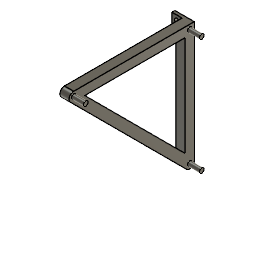
Pulley Assembly (Autodesk Fusion 360 archive; units mm, degrees)
design "Left support for pulley"
part number: 2026-04-03-14-57-29-841
Autodesk Fusion 360 part; units mm, degrees
sketch "Sketch1" plane through (0, 0, 0) normal (1, 0, 0) x (0, 1, 0)
  line L0 (171.704, 12.7) -> (-171.704, 12.7)
  line L1 (-171.704, 12.7) -> (-171.704, -12.7)
  line L2 (-171.704, -12.7) -> (171.704, -12.7)
  line L3 (171.704, -12.7) -> (171.704, 12.7)
  line L4 (171.704, 12.7) -> (-171.704, -12.7) construction
  line L5 (-171.704, 12.7) -> (171.704, -12.7) construction
  circle A0 centre (-159.004, 0) radius 12.7
  line L6 (171.704, -12.7) -> (146.304, -12.7)
  line L7 (146.304, -12.7) -> (146.304, -330.708)
  line L8 (146.304, -330.708) -> (171.704, -330.708)
  line L9 (171.704, -330.708) -> (171.704, -12.7)
  circle A1 centre (159.004, -318.008) radius 12.7
  line L10 (150.0237, -326.9883) -> (-167.9843, -8.9803)
  line L11 (150.0237, -326.9883) -> (167.9843, -309.0277)
  line L12 (150.0237, -326.9883) -> (175.4237, -326.9883) construction
  line L13 (167.9843, -309.0277) -> (-150.0237, 8.9803)
  dimension "d1" = 343.408
  dimension "d2" = 25.4
  dimension "d3" = 25.4
  dimension "d4" = 25.4
  dimension "d5" = 318.008
  dimension "d6" = 25.4
  dimension "d7" = 25.4
  dimension "d8" = 45
  constraint horizontal L0
  constraint perpendicular L0 L1
  constraint parallel L0 L2
  constraint parallel L1 L3
  constraint coincident L4 origin
  constraint coincident L5 origin
  constraint tangent L1 A0
  constraint tangent L0 A0
  constraint horizontal L6
  constraint vertical L7
  constraint horizontal L8
  constraint vertical L9
  constraint tangent L8 A1
  constraint tangent L9 A1
  constraint coincident A1 L10.start
  constraint coincident A0 L10.end
  constraint tangent A0 L10
  constraint tangent A1 L10
  constraint horizontal L12
  constraint coincident A0 L13.end
  constraint tangent A0 L13
  measures "d1" distance of L1.end L2.end
  measures "d2" distance of L0.end L1.end
  measures "d3" diameter of A0
  measures "d4" distance of L2.end L6.end
  measures "d5" distance of L2.end L8.end
  measures "d6" diameter of A1
  measures "d7" distance of L10.start L11.end
  measures "d8" angle of L11 L12
extrude "Extrude1" add sketch "Sketch1" along normal blind 25.4 contours L0 L2 L3 A0 L6 L13 | A0 | L2 L6 L7 L9 A1 L13 | L2 A0 L13 | A1 L11 | L2 L7 L10 L13 | L2 A0 L10 | L7 A1 L13 | A1 L11 | L7 A1 L10
sketch "Sketch2" plane through (0, 0, 0) normal (-1, 0, 0) x (0, -1, 0)
  line L0 (-146.304, -12.7) -> (128.3435, -12.7)
  line L1 (128.3435, -12.7) -> (-146.304, -287.3475)
  line L2 (-146.304, -287.3475) -> (-146.304, -12.7)
  line L3 (-171.704, 12.7) -> (-171.704, -318.008)
  arc A0 (-171.704, -318.008) -> (-150.0237, -326.9883) centre (-159.004, -318.008) ccw
  line L4 (-150.0237, -326.9883) -> (167.9843, -8.9803)
  arc A1 (167.9843, -8.9803) -> (159.004, 12.7) centre (159.004, 0) ccw
  line L5 (159.004, 12.7) -> (-171.704, 12.7)
  line L6 (-171.704, 12.7) -> (-163.322, 12.7)
  line L7 (-163.322, 12.7) -> (-163.322, -15.24)
  line L8 (-163.322, -15.24) -> (-171.704, -15.24)
  line L9 (-171.704, -15.24) -> (-171.704, 12.7)
  dimension "d11" = 8.382
  dimension "d12" = 27.94
  constraint horizontal L6
  constraint vertical L7
  constraint horizontal L8
  constraint vertical L9
  constraint coincident L3.start L5.end
  measures "d11" distance of L3.start L6.end
  measures "d12" distance of L3.start L8.end
extrude "Extrude2" add sketch "Sketch2" along normal blind 27.94 contours L3 L5 L6 L7 L8 L9
sketch "Sketch3" plane through (0, 163.322, 0) normal (0, -1, 0) x (1, 0, 0)
  line L0 (0, -15.24) -> (0, 12.7)
  line L1 (0, 12.7) -> (-27.94, 12.7)
  line L2 (-27.94, 12.7) -> (-27.94, -15.24)
  line L3 (-27.94, -15.24) -> (0, -15.24)
  circle A0 centre (-13.97, -1.27) radius 6.35
  dimension "d15" = 12.7
  measures "d15" diameter of A0
extrude "Extrude3" cut sketch "Sketch3" against normal blind 8.382 contours A0
sketch "Sketch4" plane through (25.4, 0, 0) normal (1, 0, 0) x (0, 1, 0)
  line L0 (-128.3435, -12.7) -> (146.304, -12.7)
  line L1 (146.304, -12.7) -> (146.304, -287.3475)
  line L2 (146.304, -287.3475) -> (-128.3435, -12.7)
  line L3 (171.704, -318.008) -> (171.704, 12.7)
  line L4 (171.704, 12.7) -> (-159.004, 12.7)
  arc A0 (-159.004, 12.7) -> (-167.9843, -8.9803) centre (-159.004, 0) ccw
  line L5 (-167.9843, -8.9803) -> (150.0237, -326.9883)
  arc A1 (150.0237, -326.9883) -> (171.704, -318.008) centre (159.004, -318.008) ccw
  circle A2 centre (-159.004, 0) radius 6.2865
  dimension "d18" = 12.573
  constraint concentric A0 A2
  measures "d18" diameter of A2
extrude "Extrude4" add sketch "Sketch4" along normal blind 33.02 contours A2
sketch "Sketch5" plane through (25.4, 0, 0) normal (1, 0, 0) x (0, 1, 0)
  circle A0 centre (-159.004, 0) radius 6.2865
  line L0 (-128.3435, -12.7) -> (146.304, -12.7)
  line L1 (146.304, -287.3475) -> (-128.3435, -12.7)
  line L2 (171.704, -318.008) -> (171.704, 12.7)
  line L3 (171.704, 12.7) -> (-159.004, 12.7)
  arc A1 (-159.004, 12.7) -> (-167.9843, -8.9803) centre (-159.004, 0) ccw
  line L4 (-167.9843, -8.9803) -> (150.0237, -326.9883)
  arc A2 (150.0237, -326.9883) -> (171.704, -318.008) centre (159.004, -318.008) ccw
  circle A3 centre (159.004, -318.008) radius 6.35
  dimension "d21" = 12.7
  constraint concentric A2 A3
  measures "d21" diameter of A3
extrude "Extrude5" add sketch "Sketch5" along normal blind 33.02 contours A3
sketch "Sketch6" plane through (25.4, 0, 0) normal (1, 0, 0) x (0, 1, 0)
  circle A0 centre (159.004, -318.008) radius 6.35
  circle A1 centre (-159.004, 0) radius 6.2865
  line L0 (-128.3435, -12.7) -> (146.304, -12.7)
  line L1 (146.304, -12.7) -> (146.304, -287.3475)
  line L2 (146.304, -287.3475) -> (-128.3435, -12.7)
  line L3 (171.704, -318.008) -> (171.704, 12.7)
  line L4 (171.704, 12.7) -> (-159.004, 12.7)
  arc A2 (-159.004, 12.7) -> (-167.9843, -8.9803) centre (-159.004, 0) ccw
  line L5 (-167.9843, -8.9803) -> (150.0237, -326.9883)
  arc A3 (150.0237, -326.9883) -> (171.704, -318.008) centre (159.004, -318.008) ccw
  line L6 (146.304, -12.7) -> (171.704, -12.7)
  line L7 (171.704, -12.7) -> (171.704, 12.7)
  line L8 (171.704, 12.7) -> (146.304, 12.7)
  line L9 (146.304, 12.7) -> (146.304, -12.7)
  circle A4 centre (159.004, 0) radius 6.35
  dimension "d24" = 12.7
  constraint horizontal L6
  constraint vertical L7
  constraint horizontal L8
  constraint vertical L9
  constraint coincident L3.end L4.start
  constraint coincident L0.end L1.start
  measures "d24" diameter of A4
extrude "Extrude6" add sketch "Sketch6" along normal blind 33.02 contours A4

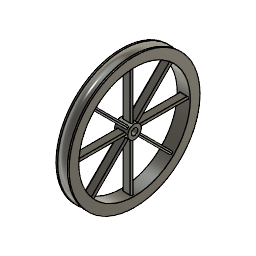
design "Pulley for the handle"
part number: 2026-04-03-13-48-15-446
Autodesk Fusion 360 part; units mm, degrees
sketch "Sketch1" plane through (0, 0, 0) normal (1, 0, 0) x (0, 1, 0)
  circle A0 centre (0, 0) radius 127
  circle A1 centre (0, 0) radius 107.95
  circle A2 centre (0, 0) radius 13.1264
  line L0 (2.8393, 12.8157) -> (2.8393, 107.9127)
  line L1 (-2.7344, 107.9154) -> (-2.7344, 12.8385)
  dimension "d1" = 254
  dimension "d2" = 215.9
  constraint coincident A0.centre A1.centre
  constraint coincident A2 L0.start
  constraint coincident A1 L0.end
  constraint vertical L0
  constraint coincident A1 L1.start
  constraint coincident A2 L1.end
  constraint parallel L0 L1
  measures "d1" diameter of A0
  measures "d2" diameter of A1
extrude "Extrude1" add sketch "Sketch1" along normal blind 19.05 contours A1 A2 L0 L1 picked at (0.3629, 44.7105) makes body 1
pattern_circular "C-Pattern1" count 8 over 360 about axis through (1.75, 0, 0) along (1, 0, 0) of bodies 1 makes body 2 at (6.35, -29.4689, 33.4843) makes body 3 at (12.7, -44.5147, 2.8393) makes body 4 at (6.35, -33.4843, -29.4689) makes body 5 at (12.7, -2.8393, -44.5147) makes body 6 at (6.35, 29.4689, -33.4843) makes body 7 at (12.7, 44.5147, -2.8393) makes body 8 at (6.35, 33.4843, 29.4689)
move_body "Move1" bodies 3 2 4 1 8 5 6 7 to x (1, 0, 0) y (0, 1, 0) z (0, 0, 1) at (3.175, 0, 0)
sketch "Sketch2" plane through (0, 0, 0) normal (1, 0, 0) x (0, 1, 0)
  circle A0 centre (0, 0) radius 13.2274
  circle A1 centre (0, 0) radius 107.95
  circle A2 centre (0, 0) radius 127
  constraint coincident A0.centre A1.centre
  constraint concentric A0 A1
  constraint concentric A1 A2
extrude "Extrude2" add sketch "Sketch2" along normal blind 25.4 bodies 1 2 3 4 5 6 7 8
sketch "Sketch3" plane through (0, 0, 0) normal (-1, 0, 0) x (0, -1, 0)
  circle A0 centre (0, 0) radius 13.2274
  circle A1 centre (0, 0) radius 6.35
  constraint concentric A0 A1
extrude "Extrude3" cut sketch "Sketch3" against normal blind 25.4 contours A1 bodies 1
sketch "Sketch4" plane through (0, 0, 0) normal (0, 1, 0) x (1, 0, 0)
  circle A0 centre (12.7, -127) radius 9.525
  dimension "d11" = 19.05
  measures "d11" diameter of A0
sketch "Sketch5" plane through (0, 0, 0) normal (1, 0, 0) x (0, 1, 0)
  circle A0 centre (0, 0) radius 127
  constraint coincident A0.centre origin
sweep "Sweep1" cut profiles "Sketch4" path "Sketch5" along A0 section 1 bodies 1
fillet "Fillet1" radius 2.7864 4 edges at (22.225, 2.8393, 60.4159) (22.225, -2.7344, 60.4285) (3.175, -2.7344, 60.4285) (3.175, 2.8393, 60.4159) on bodies 1
fillet "Fillet2" radius 2.7864 28 edges at (3.175, -44.6629, 40.7959) (3.175, -40.7127, 44.7282) (22.225, -40.7127, 44.7282) (22.225, -44.6629, 40.7959) (3.175, -60.4285, -2.7344) (22.225, -60.4159, 2.8393) (3.175, -60.4159, 2.8393) (22.225, -60.4285, -2.7344) (22.225, -44.7282, -40.7127) (3.175, -44.7282, -40.7127) (22.225, -40.7959, -44.6629) (3.175, -40.7959, -44.6629) (22.225, -2.8393, -60.4159) (22.225, 2.7344, -60.4285) (3.175, -2.8393, -60.4159) (3.175, 2.7344, -60.4285) (22.225, 40.7127, -44.7282) (22.225, 44.6629, -40.7959) (3.175, 40.7127, -44.7282) (3.175, 44.6629, -40.7959) (22.225, 60.4159, -2.8393) (22.225, 60.4285, 2.7344) (3.175, 60.4159, -2.8393) (3.175, 60.4285, 2.7344) (22.225, 40.7959, 44.6629) (22.225, 44.7282, 40.7127) (3.175, 40.7959, 44.6629) (3.175, 44.7282, 40.7127) on bodies 1

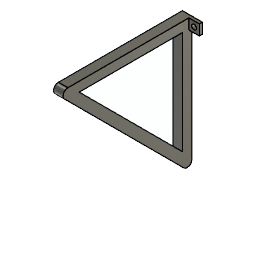
design "Right Support for Pulley"
part number: 2026-04-03-13-47-48-365
Autodesk Fusion 360 part; units mm, degrees
sketch "Sketch1" plane through (0, 0, 0) normal (1, 0, 0) x (0, 1, 0)
  line L0 (171.704, 12.7) -> (-171.704, 12.7)
  line L1 (-171.704, 12.7) -> (-171.704, -12.7)
  line L2 (-171.704, -12.7) -> (171.704, -12.7)
  line L3 (171.704, -12.7) -> (171.704, 12.7)
  line L4 (171.704, 12.7) -> (-171.704, -12.7) construction
  line L5 (-171.704, 12.7) -> (171.704, -12.7) construction
  circle A0 centre (-159.004, 0) radius 12.7
  line L6 (171.704, -12.7) -> (146.304, -12.7)
  line L7 (146.304, -12.7) -> (146.304, -330.708)
  line L8 (146.304, -330.708) -> (171.704, -330.708)
  line L9 (171.704, -330.708) -> (171.704, -12.7)
  circle A1 centre (159.004, -318.008) radius 12.7
  line L10 (-171.704, -5.2605) -> (150.0237, -326.9883)
  line L11 (-171.704, -5.2605) -> (-153.7435, 12.7)
  line L12 (-171.704, -5.2605) -> (-146.304, -5.2605) construction
  line L13 (-153.7435, 12.7) -> (170.7899, -311.8334)
  dimension "d1" = 343.408
  dimension "d2" = 25.4
  dimension "d3" = 25.4
  dimension "d4" = 318.008
  dimension "d5" = 25.4
  dimension "d6" = 45
  dimension "d7" = 25.4
  constraint horizontal L0
  constraint perpendicular L0 L1
  constraint parallel L0 L2
  constraint parallel L1 L3
  constraint coincident L4 origin
  constraint coincident L5 origin
  constraint tangent L1 A0
  constraint tangent L0 A0
  constraint horizontal L6
  constraint vertical L7
  constraint horizontal L8
  constraint vertical L9
  constraint tangent L8 A1
  constraint tangent L9 A1
  constraint coincident L1 L10.start
  constraint coincident A1 L10.end
  constraint tangent A1 L10
  constraint horizontal L12
  constraint perpendicular L10 L11
  constraint tangent A1 L13
  measures "d1" distance of L1.end L2.end
  measures "d2" distance of L0.end L1.end
  measures "d3" distance of L2.end L6.end
  measures "d4" distance of L2.end L8.end
  measures "d5" diameter of A1
  measures "d6" angle of L11 L12
  measures "d7" distance of L10.start L11.end
extrude "Extrude1" add sketch "Sketch1" along normal blind 25.4 contours L0 L2 L3 L6 L13 | L0 A0 L11 | A0 L11 L13 | L2 L6 L7 L9 A1 L13 | A0 L11 | A0 L11 | L2 A0 L13 | A1 | L2 L7 L10 L13 | L7 A1 L13 | L2 A0 L10 | L7 A1 L10
sketch "Sketch2" plane through (25.4, 0, 0) normal (1, 0, 0) x (0, 1, 0)
  line L0 (146.304, -287.3475) -> (-128.3435, -12.7)
  line L1 (-128.3435, -12.7) -> (146.304, -12.7)
  line L2 (146.304, -12.7) -> (146.304, -287.3475)
  arc A0 (-159.004, 12.7) -> (-167.9843, -8.9803) centre (-159.004, 0) ccw
  line L3 (-167.9843, -8.9803) -> (150.0237, -326.9883)
  arc A1 (150.0237, -326.9883) -> (171.704, -318.008) centre (159.004, -318.008) ccw
  line L4 (171.704, -318.008) -> (171.704, 12.7)
  line L5 (171.704, 12.7) -> (-159.004, 12.7)
  line L6 (171.704, 12.7) -> (163.322, 12.7)
  line L7 (163.322, 12.7) -> (163.322, -15.24)
  line L8 (163.322, -15.24) -> (171.704, -15.24)
  line L9 (171.704, -15.24) -> (171.704, 12.7)
  dimension "d10" = 8.382
  dimension "d11" = 27.94
  constraint horizontal L6
  constraint vertical L7
  constraint horizontal L8
  constraint vertical L9
  constraint coincident L4.end L5.start
  measures "d10" distance of L4.end L6.end
  measures "d11" distance of L4.end L8.end
extrude "Extrude2" add sketch "Sketch2" along normal blind 27.94 contours L4 L5 L6 L7 L8 L9
sketch "Sketch3" plane through (0, 163.322, 0) normal (0, -1, 0) x (1, 0, 0)
  line L0 (25.4, 12.7) -> (25.4, -15.24)
  line L1 (25.4, -15.24) -> (53.34, -15.24)
  line L2 (53.34, -15.24) -> (53.34, 12.7)
  line L3 (53.34, 12.7) -> (25.4, 12.7)
  circle A0 centre (39.37, -1.27) radius 6.35
  dimension "d14" = 27.94
  dimension "d15" = 27.94
  dimension "d16" = 12.7
  measures "d14" distance of L0.start L2.end
  measures "d15" distance of L1.end L2.end
  measures "d16" diameter of A0
extrude "Extrude3" cut sketch "Sketch3" against normal blind 8.382 contours A0
sketch "Sketch4" plane through (0, 0, 0) normal (-1, 0, 0) x (0, -1, 0)
  line L0 (128.3435, -12.7) -> (-146.304, -287.3475)
  line L1 (-146.304, -287.3475) -> (-146.304, -12.7)
  line L2 (-146.304, -12.7) -> (128.3435, -12.7)
  arc A0 (167.9843, -8.9803) -> (159.004, 12.7) centre (159.004, 0) ccw
  line L3 (159.004, 12.7) -> (-171.704, 12.7)
  line L4 (-171.704, 12.7) -> (-171.704, -318.008)
  arc A1 (-171.704, -318.008) -> (-150.0237, -326.9883) centre (-159.004, -318.008) ccw
  line L5 (-150.0237, -326.9883) -> (167.9843, -8.9803)
sketch "Sketch5" plane through (0, 0, 0) normal (-1, 0, 0) x (0, -1, 0)
  circle A0 centre (-158.75, 0) radius 6.4135
  circle A1 centre (-158.6956, -318.008) radius 6.4135
  circle A2 centre (159.004, 0) radius 6.35
  arc A3 (167.9843, -8.9803) -> (159.004, 12.7) centre (159.004, 0) ccw
  line L0 (159.004, 12.7) -> (159.004, 0)
  line L1 (-171.704, -318.008) -> (-148.59, -318.008)
  dimension "d19" = 12.827
  dimension "d20" = 12.827
  dimension "d21" = 12.7
  dimension "d22" = 12.7
  constraint coincident A2.centre A3.centre
  constraint coincident A3.end L0.start
  constraint horizontal L1
  constraint coincident A1.centre L1
  measures "d19" diameter of A0
  measures "d20" diameter of A1
  measures "d21" diameter of A2
  measures "d22" radius of A3
extrude "Extrude4" cut sketch "Sketch5" against normal blind 5.08
